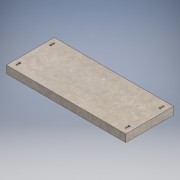
# Autodesk Inventor part: B soffit
Saved by Autodesk Inventor 2022.2 (Build 262287010, 287A)
## iProperties
Created: 2022-01-21
Part Number: B soffit
Material: Limestone
Document SubType Name: Modeling
Designer: awelt
Density: 2.6 g/cm^3
Appearance: Kasota Gray
Mass: 114869 g
Surface Area: 14352.5 cm^2
Volume: 44180.5 cm^3
Author: awelt
Autodesk Inventor part; units mm, degrees
ref_plane "YZ Plane" through (0, 0, 0) normal (1, 0, 0) x (0, 1, 0)
ref_plane "XZ Plane" through (0, 0, 0) normal (0, 1, 0) x (-1, 0, 0)
ref_plane "XY Plane" through (0, 0, 0) normal (0, 0, 1) x (1, 0, 0)
sketch "Bolt" plane through (0, 0, 0) normal (0, 0, 1) x (1, 0, 0)
  line L0 (25.0072, -4.4715) -> (29.7779, -8.6)
  line L1 (-7.366, -4.2392) -> (24.384, -4.2392)
  arc A0 (25.0072, -4.4715) -> (24.384, -4.2392) centre (24.384, -5.1917) ccw
  arc A1 (32.8161, -7.341) -> (33.3155, 0.6503) centre (-19.0704, -0.0877) ccw
  arc A2 (29.6829, -8.5178) -> (32.8161, -7.341) centre (30.9295, -7.0773) ccw
  line L2 (-7.366, -4.2392) -> (-7.366, 0.6503)
  line L3 (-7.366, 5.5398) -> (-7.366, 0.6503)
  line L4 (-7.366, 5.5398) -> (24.384, 5.5398)
  arc A3 (24.384, 5.5398) -> (25.0072, 5.772) centre (24.384, 6.4923) ccw
  line L5 (25.0072, 5.772) -> (29.7779, 9.9005)
  arc A4 (32.8161, 8.6415) -> (29.6829, 9.8183) centre (30.9295, 8.3778) ccw
  arc A5 (33.3155, 0.6503) -> (32.8161, 8.6415) centre (-19.0704, 1.3882) ccw
  dimension "d2" = 1203.325
sketch "Block2" plane through (0, 0, 0) normal (0, 0, 1) x (1, 0, 0)
  line L0 (55.9218, 83.1733) -> (60.0503, 87.944)
  line L1 (55.6895, 50.8) -> (55.6895, 82.55)
  arc A0 (55.9218, 83.1733) -> (55.6895, 82.55) centre (56.642, 82.55) ccw
  arc A1 (58.7912, 90.9822) -> (50.8, 91.4815) centre (51.5379, 39.0956) ccw
  arc A2 (59.968, 87.8489) -> (58.7912, 90.9822) centre (58.5275, 89.0955) ccw
  line L2 (55.6895, 50.8) -> (50.8, 50.8)
  line L3 (45.9105, 50.8) -> (50.8, 50.8)
  line L4 (45.9105, 50.8) -> (45.9105, 82.55)
  arc A3 (45.9105, 82.55) -> (45.6782, 83.1733) centre (44.958, 82.55) ccw
  line L5 (45.6782, 83.1733) -> (41.5497, 87.944)
  arc A4 (42.8088, 90.9822) -> (41.632, 87.8489) centre (43.0725, 89.0955) ccw
  arc A5 (50.8, 91.4815) -> (42.8088, 90.9822) centre (50.0621, 39.0956) ccw
  point P0 (50.8, 50.8)
  dimension "d2" = 1203.325
sketch "Block3" plane through (0, 0, 0) normal (0, 0, 1) x (1, 0, 0)
  line L0 (958.063, 109.0167) -> (953.9345, 104.246)
  line L1 (958.2953, 141.3899) -> (958.2953, 109.6399)
  arc A0 (958.063, 109.0167) -> (958.2953, 109.6399) centre (957.3428, 109.6399) ccw
  arc A1 (955.1935, 101.2078) -> (963.1848, 100.7084) centre (962.4468, 153.0943) ccw
  arc A2 (954.0168, 104.341) -> (955.1935, 101.2078) centre (955.4573, 103.0944) ccw
  line L2 (958.2953, 141.3899) -> (963.1848, 141.3899)
  line L3 (968.0743, 141.3899) -> (963.1848, 141.3899)
  line L4 (968.0743, 141.3899) -> (968.0743, 109.6399)
  arc A3 (968.0743, 109.6399) -> (968.3065, 109.0167) centre (969.0268, 109.6399) ccw
  line L5 (968.3065, 109.0167) -> (972.435, 104.246)
  arc A4 (971.176, 101.2078) -> (972.3528, 104.341) centre (970.9123, 103.0944) ccw
  arc A5 (963.1848, 100.7084) -> (971.176, 101.2078) centre (963.9227, 153.0943) ccw
  point P0 (963.1848, 141.3899)
  dimension "d2" = 1203.325
sketch "Sketch1" plane through (0, 0, 0) normal (1, 0, 0) x (0, 1, 0)
  line L0 (0, 0) -> (50.8, 0)
  line L1 (50.8, 0) -> (50.8, 482.6)
  line L2 (50.8, 482.6) -> (0, 482.6)
  line L3 (0, 482.6) -> (0, 0) construction
  line L4 (0, 482.6) -> (-25.4, 482.6)
  line L5 (-25.4, 482.6) -> (-25.4, 0)
  line L6 (-25.4, 0) -> (0, 0)
  dimension "d0" = 50.8
  dimension "d1" = 482.6
  dimension "d5" = 25.4
  constraints: 14 end point, 3 perpendicular, 2 horizontal, 2 parallel
  measures "d0" distance of L2.end L1.end
  measures "d1" distance of L1.end L0.end
  measures "d5" distance of L2.end L4.end
extrude "Extrusion1" add sketch "Sketch1" along normal blind 1203.325
sketch "Sketch2" plane through (0, 50.8, 482.6) normal (0, 1, 0) x (1, 0, 0)
  line L0 (0, 482.6) -> (0, 0) projected
  line L1 (0, 0) -> (1203.325, 0) projected
  line L2 (1203.325, 482.6) -> (1203.325, 0) projected
  line L3 (0, 482.6) -> (1203.325, 482.6) projected
  line L4 (1152.525, 431.8) -> (1152.525, 50.8) construction
  line L5 (1152.525, 50.8) -> (50.8, 50.8) construction
  line L6 (50.8, 50.8) -> (50.8, 431.8) construction
  line L7 (50.8, 431.8) -> (1152.525, 431.8) construction
  line L8 (1152.525, 431.8) -> (1152.525, 391.1185)
  line L9 (50.8, 431.8) -> (50.8, 391.1185)
  line L10 (50.8, 50.8) -> (50.8, 91.4815)
  line L11 (1152.525, 50.8) -> (1152.525, 91.4815)
  line L12 (55.9218, 83.1733) -> (60.0503, 87.944)
  line L13 (55.6895, 50.8) -> (55.6895, 82.55)
  arc A0 (55.9218, 83.1733) -> (55.6895, 82.55) centre (56.642, 82.55) ccw
  arc A1 (58.7912, 90.9822) -> (50.8, 91.4815) centre (51.5379, 39.0956) ccw
  arc A2 (59.968, 87.8489) -> (58.7912, 90.9822) centre (58.5275, 89.0955) ccw
  line L14 (55.6895, 50.8) -> (50.8, 50.8)
  line L15 (45.9105, 50.8) -> (50.8, 50.8)
  line L16 (45.9105, 50.8) -> (45.9105, 82.55)
  arc A3 (45.9105, 82.55) -> (45.6782, 83.1733) centre (44.958, 82.55) ccw
  line L17 (45.6782, 83.1733) -> (41.5497, 87.944)
  arc A4 (42.8088, 90.9822) -> (41.632, 87.8489) centre (43.0725, 89.0955) ccw
  arc A5 (50.8, 91.4815) -> (42.8088, 90.9822) centre (50.0621, 39.0956) ccw
  line L18 (1157.6468, 83.1733) -> (1161.7753, 87.944)
  line L19 (1157.4145, 50.8) -> (1157.4145, 82.55)
  arc A6 (1157.6468, 83.1733) -> (1157.4145, 82.55) centre (1158.367, 82.55) ccw
  arc A7 (1160.5162, 90.9822) -> (1152.525, 91.4815) centre (1153.2629, 39.0956) ccw
  arc A8 (1161.693, 87.8489) -> (1160.5162, 90.9822) centre (1160.2525, 89.0955) ccw
  line L20 (1157.4145, 50.8) -> (1152.525, 50.8)
  line L21 (1147.6355, 50.8) -> (1152.525, 50.8)
  line L22 (1147.6355, 50.8) -> (1147.6355, 82.55)
  arc A9 (1147.6355, 82.55) -> (1147.4032, 83.1733) centre (1146.683, 82.55) ccw
  line L23 (1147.4032, 83.1733) -> (1143.2747, 87.944)
  arc A10 (1144.5338, 90.9822) -> (1143.357, 87.8489) centre (1144.7975, 89.0955) ccw
  arc A11 (1152.525, 91.4815) -> (1144.5338, 90.9822) centre (1151.7871, 39.0956) ccw
  line L24 (1147.4032, 399.4267) -> (1143.2747, 394.656)
  line L25 (1147.6355, 431.8) -> (1147.6355, 400.05)
  arc A12 (1147.4032, 399.4267) -> (1147.6355, 400.05) centre (1146.683, 400.05) ccw
  arc A13 (1144.5338, 391.6178) -> (1152.525, 391.1185) centre (1151.7871, 443.5044) ccw
  arc A14 (1143.357, 394.7511) -> (1144.5338, 391.6178) centre (1144.7975, 393.5045) ccw
  line L26 (1147.6355, 431.8) -> (1152.525, 431.8)
  line L27 (1157.4145, 431.8) -> (1152.525, 431.8)
  line L28 (1157.4145, 431.8) -> (1157.4145, 400.05)
  arc A15 (1157.4145, 400.05) -> (1157.6468, 399.4267) centre (1158.367, 400.05) ccw
  line L29 (1157.6468, 399.4267) -> (1161.7753, 394.656)
  arc A16 (1160.5162, 391.6178) -> (1161.693, 394.7511) centre (1160.2525, 393.5045) ccw
  arc A17 (1152.525, 391.1185) -> (1160.5162, 391.6178) centre (1153.2629, 443.5044) ccw
  line L30 (45.6782, 399.4267) -> (41.5497, 394.656)
  line L31 (45.9105, 431.8) -> (45.9105, 400.05)
  arc A18 (45.6782, 399.4267) -> (45.9105, 400.05) centre (44.958, 400.05) ccw
  arc A19 (42.8088, 391.6178) -> (50.8, 391.1185) centre (50.0621, 443.5044) ccw
  arc A20 (41.632, 394.7511) -> (42.8088, 391.6178) centre (43.0725, 393.5045) ccw
  line L32 (45.9105, 431.8) -> (50.8, 431.8)
  line L33 (55.6895, 431.8) -> (50.8, 431.8)
  line L34 (55.6895, 431.8) -> (55.6895, 400.05)
  arc A21 (55.6895, 400.05) -> (55.9218, 399.4267) centre (56.642, 400.05) ccw
  line L35 (55.9218, 399.4267) -> (60.0503, 394.656)
  arc A22 (58.7912, 391.6178) -> (59.968, 394.7511) centre (58.5275, 393.5045) ccw
  arc A23 (50.8, 391.1185) -> (58.7912, 391.6178) centre (51.5379, 443.5044) ccw
  point P0 (45.6782, 83.1733)
  point P1 (50.8, 50.8)
  point P2 (55.6895, 50.8)
  point P3 (55.6895, 82.55)
  point P4 (55.9218, 83.1733)
  point P5 (59.968, 87.8489)
  point P6 (58.7912, 90.9822)
  point P7 (50.8, 91.4815)
  point P8 (42.8088, 90.9822)
  point P9 (41.632, 87.8489)
  point P10 (1157.4145, 82.55)
  point P11 (1157.6468, 83.1733)
  point P12 (1160.5162, 90.9822)
  point P13 (1152.525, 91.4815)
  point P14 (1144.5338, 90.9822)
  point P15 (1147.4032, 83.1733)
  point P16 (1147.6355, 82.55)
  point P17 (1147.6355, 50.8)
  point P18 (1152.525, 50.8)
  point P19 (1157.4145, 50.8)
  point P20 (45.9105, 400.05)
  point P21 (45.6782, 399.4267)
  point P22 (41.632, 394.7511)
  point P23 (42.8088, 391.6178)
  point P24 (50.8, 391.1185)
  point P25 (58.7912, 391.6178)
  point P26 (59.968, 394.7511)
  point P27 (55.9218, 399.4267)
  point P28 (55.6895, 400.05)
  point P29 (55.6895, 431.8)
  point P30 (50.8, 431.8)
  point P31 (45.9105, 431.8)
  point P32 (1157.6468, 399.4267)
  point P33 (1157.4145, 400.05)
  point P34 (1157.4145, 431.8)
  point P35 (1152.525, 431.8)
  point P36 (1147.6355, 431.8)
  point P37 (1147.6355, 400.05)
  point P38 (1147.4032, 399.4267)
  point P39 (1143.357, 394.7511)
  point P40 (1144.5338, 391.6178)
  point P41 (1152.525, 391.1185)
  point P42 (1160.5162, 391.6178)
  point P43 (1161.693, 394.7511)
  dimension "d2" = 1203.325
  dimension "d4" = 50.8
  constraints: 16 end point, 3 collinear, 1 vertical, 15 other
  measures "d4" distance between parallel lines of L3 L7
revolve "Revolution1" cut sketch "Sketch2" angle 90 about axis through (1152.525, 50.8, 431.8) along (-1, 0, 0) contours L15 L16 A3 L17 A4 A5 L10 | L10 A1 A2 L12 A0 L13 L14 | L21 L22 A9 L23 A10 A11 L11 | L11 A7 A8 L18 A6 L19 L20
revolve "Revolution2" cut sketch "Sketch2" angle 90 about axis through (50.8, 50.8, 50.8) along (1, 0, 0) contours L27 L28 A15 L29 A16 A17 L8 | L8 A13 A14 L24 A12 L25 L26 | L33 L34 A21 L35 A22 A23 L9 | L9 A19 A20 L30 A18 L31 L32
sketch "Sketch3" plane through (45.9105, 50.8, 50.8) normal (0, 0, 1) x (1, 0, 0)
  line L0 (1106.6145, 0) -> (1106.6145, 2.2959)
  line L1 (4.8895, 0) -> (4.8895, 1.0294)
  line L2 (4.8895, 0) -> (4.8895, -40.6815)
  line L3 (1106.6145, 0) -> (1106.6145, -40.6815)
  line L4 (-0.2323, -32.3733) -> (-4.3608, -37.144)
  line L5 (0, 0) -> (0, -31.75)
  arc A0 (-0.2323, -32.3733) -> (0, -31.75) centre (-0.9525, -31.75) ccw
  arc A1 (-3.1017, -40.1822) -> (4.8895, -40.6815) centre (4.1516, 11.7044) ccw
  arc A2 (-4.2785, -37.0489) -> (-3.1017, -40.1822) centre (-2.838, -38.2955) ccw
  line L6 (0, 0) -> (4.8895, 0)
  line L7 (9.779, 0) -> (4.8895, 0)
  line L8 (9.779, 0) -> (9.779, -31.75)
  arc A3 (9.779, -31.75) -> (10.0113, -32.3733) centre (10.7315, -31.75) ccw
  line L9 (10.0113, -32.3733) -> (14.1398, -37.144)
  arc A4 (12.8807, -40.1822) -> (14.0575, -37.0489) centre (12.617, -38.2955) ccw
  arc A5 (4.8895, -40.6815) -> (12.8807, -40.1822) centre (5.6274, 11.7044) ccw
  line L10 (1101.4927, -32.3733) -> (1097.3642, -37.144)
  line L11 (1101.725, 0) -> (1101.725, -31.75)
  arc A6 (1101.4927, -32.3733) -> (1101.725, -31.75) centre (1100.7725, -31.75) ccw
  arc A7 (1098.6233, -40.1822) -> (1106.6145, -40.6815) centre (1105.8766, 11.7044) ccw
  arc A8 (1097.4465, -37.0489) -> (1098.6233, -40.1822) centre (1098.887, -38.2955) ccw
  line L12 (1101.725, 0) -> (1106.6145, 0)
  line L13 (1111.504, 0) -> (1106.6145, 0)
  line L14 (1111.504, 0) -> (1111.504, -31.75)
  arc A9 (1111.504, -31.75) -> (1111.7363, -32.3733) centre (1112.4565, -31.75) ccw
  line L15 (1111.7363, -32.3733) -> (1115.8648, -37.144)
  arc A10 (1114.6057, -40.1822) -> (1115.7825, -37.0489) centre (1114.342, -38.2955) ccw
  arc A11 (1106.6145, -40.6815) -> (1114.6057, -40.1822) centre (1107.3524, 11.7044) ccw
  point P0 (-45.9105, -50.8)
  point P1 (4.8895, 0)
  point P2 (1106.6145, 0)
  point P3 (4.8895, -40.6815)
  point P4 (12.8807, -40.1822)
  point P5 (14.0575, -37.0489)
  point P6 (10.0113, -32.3733)
  point P7 (9.779, -31.75)
  point P8 (9.779, 0)
  point P9 (4.8895, 0)
  point P10 (1106.6145, -40.6815)
  point P11 (1114.6057, -40.1822)
  point P12 (1115.7825, -37.0489)
  point P13 (1111.7363, -32.3733)
  point P14 (1111.504, -31.75)
  point P15 (1111.504, 0)
  dimension "d2" = 1203.325
  constraints: 8 end point, 4 vertical, 6 other
revolve "Revolution3" cut sketch "Sketch3" angle 360 about axis through (50.8, 50.8, 50.8) along (0, -1, 0) contours L7 L8 A3 L9 A4 A5 L2
revolve "Revolution4" cut sketch "Sketch3" angle 360 about axis through (1152.525, 50.8, 50.8) along (0, -1, 0) contours L13 L14 A9 L15 A10 A11 L3
sketch "Sketch4" plane through (1157.4145, 50.8, 431.8) normal (0, 0, -1) x (-1, 0, 0)
  line L0 (4.8895, 0) -> (4.8895, -40.6815)
  line L1 (1106.6145, 0) -> (1106.6145, -40.6815)
  line L2 (-0.2323, -32.3733) -> (-4.3608, -37.144)
  line L3 (0, 0) -> (0, -31.75)
  arc A0 (-0.2323, -32.3733) -> (0, -31.75) centre (-0.9525, -31.75) ccw
  arc A1 (-3.1017, -40.1822) -> (4.8895, -40.6815) centre (4.1516, 11.7044) ccw
  arc A2 (-4.2785, -37.0489) -> (-3.1017, -40.1822) centre (-2.838, -38.2955) ccw
  line L4 (0, 0) -> (4.8895, 0)
  line L5 (9.779, 0) -> (4.8895, 0)
  line L6 (9.779, 0) -> (9.779, -31.75)
  arc A3 (9.779, -31.75) -> (10.0113, -32.3733) centre (10.7315, -31.75) ccw
  line L7 (10.0113, -32.3733) -> (14.1398, -37.144)
  arc A4 (12.8807, -40.1822) -> (14.0575, -37.0489) centre (12.617, -38.2955) ccw
  arc A5 (4.8895, -40.6815) -> (12.8807, -40.1822) centre (5.6274, 11.7044) ccw
  line L8 (1101.4927, -32.3733) -> (1097.3642, -37.144)
  line L9 (1101.725, 0) -> (1101.725, -31.75)
  arc A6 (1101.4927, -32.3733) -> (1101.725, -31.75) centre (1100.7725, -31.75) ccw
  arc A7 (1098.6233, -40.1822) -> (1106.6145, -40.6815) centre (1105.8766, 11.7044) ccw
  arc A8 (1097.4465, -37.0489) -> (1098.6233, -40.1822) centre (1098.887, -38.2955) ccw
  line L10 (1101.725, 0) -> (1106.6145, 0)
  line L11 (1111.504, 0) -> (1106.6145, 0)
  line L12 (1111.504, 0) -> (1111.504, -31.75)
  arc A9 (1111.504, -31.75) -> (1111.7363, -32.3733) centre (1112.4565, -31.75) ccw
  line L13 (1111.7363, -32.3733) -> (1115.8648, -37.144)
  arc A10 (1114.6057, -40.1822) -> (1115.7825, -37.0489) centre (1114.342, -38.2955) ccw
  arc A11 (1106.6145, -40.6815) -> (1114.6057, -40.1822) centre (1107.3524, 11.7044) ccw
  point P0 (1157.4145, -50.8)
  point P1 (1106.6145, 0)
  point P2 (4.8895, 0)
  point P3 (1111.7363, -32.3733)
  point P4 (1111.504, -31.75)
  point P5 (1111.504, 0)
  point P6 (1106.6145, 0)
  point P7 (1106.6145, -40.6815)
  point P8 (1114.6057, -40.1822)
  point P9 (1115.7825, -37.0489)
  point P10 (10.0113, -32.3733)
  point P11 (9.779, -31.75)
  point P12 (9.779, 0)
  point P13 (4.8895, 0)
  point P14 (4.8895, -40.6815)
  point P15 (12.8807, -40.1822)
  point P16 (14.0575, -37.0489)
  dimension "d2" = 1203.325
  constraints: 4 end point, 2 vertical, 6 other
revolve "Revolution5" cut sketch "Sketch4" angle 360 about axis through (50.8, 50.8, 431.8) along (0, -1, 0) contours L11 L12 A9 L13 A10 A11 L1
revolve "Revolution6" cut sketch "Sketch4" angle 360 about axis through (1152.525, 50.8, 431.8) along (0, -1, 0) contours L5 L6 A3 L7 A4 A5 L0
body "Solid1"
